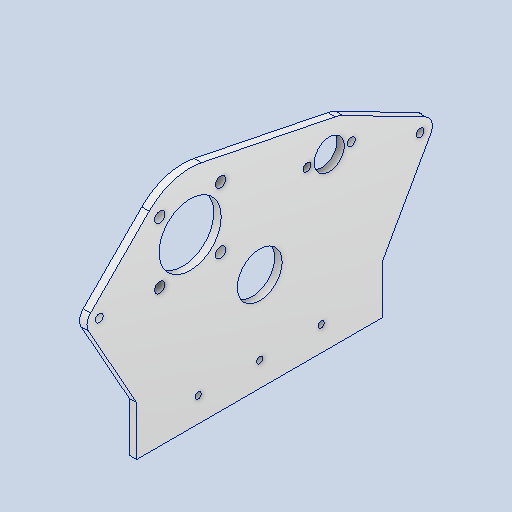
# Autodesk Inventor part: base_weel-v3-Plate-2
Saved by Autodesk Inventor 2025.2 (Build 292293000, 293)
## iProperties
Created: 2025-04-01
Part Number: base_weel-v3-Plate-2
Material: アルミニウム 6061
Document SubType Name: Modeling
Designer: haruy
Density: 2.7 g/cm^3
Appearance: アルミニウム - フラット
Author: haruy
Autodesk Inventor part; units mm, degrees
ref_plane "YZ Plane" through (0, 0, 0) normal (1, 0, 0) x (0, 1, 0)
ref_plane "XZ Plane" through (0, 0, 0) normal (0, 1, 0) x (-1, 0, 0)
ref_plane "XY Plane" through (0, 0, 0) normal (0, 0, 1) x (1, 0, 0)
derived "base_weel-v3-Plate-1.ipt"
sketch "スケッチ1" plane through (0, 0, 0) normal (1, 0, 0) x (0, 1, 0)
  line L0 (0, 0) -> (20, 0)
  line L1 (20, 0) -> (20, -110)
  line L2 (20, -110) -> (0, -110)
  line L3 (0, -110) -> (0, 0)
  circle A0 centre (40, -55) radius 52.5
  line L4 (-12.5, 72.5213) -> (-12.5, -343.3137)
  circle A1 centre (40, -55) radius 9.5 construction
  circle A2 centre (40, -55) radius 20
  circle A3 centre (68.2843, -26.7157) radius 20
  circle A4 centre (68.2843, -83.2843) radius 20
  line L5 (68.2843, -26.7157) -> (40, -55)
  line L6 (40, -55) -> (68.2843, -83.2843)
  line L7 (40, -55) -> (40, -2.5)
  line L8 (0, 15) -> (20, 15)
  line L9 (20, 15) -> (20, -125)
  line L10 (20, -125) -> (0, -125)
  line L11 (0, -125) -> (0, 15)
  circle A5 centre (68.2843, -26.7157) radius 23.5
  circle A6 centre (57.4091, 10.2164) radius 5
  circle A7 centre (57.4091, -120.2164) radius 5
  line L12 (20, -20) -> (0, -20)
  line L13 (0, -55) -> (20, -55)
  circle A8 centre (40, -55) radius 9.1
  circle A9 centre (57.4091, 10.2164) radius 1.6
  circle A10 centre (57.4091, -120.2164) radius 1.6
  line L14 (20, -20) -> (53.8799, 13.7583)
  line L15 (62.4057, 10.0326) -> (59.9865, -55.7352)
  circle A11 centre (10, -55) radius 1.25
  circle A12 centre (10, -35) radius 1.25 construction
  line L16 (62.4057, -120.0326) -> (59.9865, -54.2648)
  line L17 (20, -90) -> (53.8799, -123.7583)
  circle A13 centre (10, -75) radius 1.25 construction
  line L18 (20, -90) -> (0, -90)
  line L19 (20, -5) -> (0, -5)
  circle A14 centre (10, -30) radius 1.25
  circle A15 centre (68.2843, -26.7157) radius 12.6
  circle A16 centre (68.2843, -26.7157) radius 17.5
  circle A17 centre (80.6586, -14.3414) radius 2.1
  line L20 (68.2843, -26.7157) -> (68.2843, -9.2157)
  line L21 (68.2843, -26.7157) -> (80.6586, -14.3414)
  circle A18 centre (55.9099, -14.3414) radius 2.1
  circle A19 centre (55.9099, -39.0901) radius 2.1
  circle A20 centre (80.6586, -39.0901) radius 2.1
  circle A21 centre (68.2843, -83.2843) radius 6.1
  circle A22 centre (68.2843, -83.2843) radius 9
  circle A23 centre (68.2843, -74.2843) radius 1.6
  line L22 (68.2843, -83.2843) -> (68.2843, -74.2843)
  line L23 (20, -5) -> (54.9662, 14.579)
  line L24 (60.9367, 13.7597) -> (84.8644, -10.0619)
  circle A24 centre (68.2843, -83.2843) radius 12.25
  circle A25 centre (68.2843, -92.2843) radius 1.6
  line L25 (91.3149, -31.3893) -> (80.2896, -85.7205)
  line L26 (61.8537, -122.5067) -> (79.1735, -88.8955)
  line L27 (20, -105) -> (0, -105)
  circle A26 centre (10, -80) radius 1.25
  line L28 (20, -105) -> (54.9662, -124.579)
  point P0 (58.8173, -48.2245)
  point P1 (60.2417, -48.7967)
  point P2 (60.6843, -36.7656)
  point P3 (60.4778, -42.3781)
  point P4 (57.4812, -40.4833)
  point P5 (57.3948, -37.6052)
  point P6 (59.3747, -35.6253)
  point P7 (0.8688, -20)
  point P8 (0, -20.9963)
  point P9 (0, -89.0037)
  point P10 (0.8688, -90)
  point P11 (0, -90)
  point P12 (0, -105)
  point P13 (89.8597, -38.5603)
  point P14 (89.359, -37.1131)
  point P15 (0, -5)
  point P16 (0, -20)
  point P17 (60.0135, -55)
  dimension "d14" = 18
  dimension "d1" = 20
  dimension "d2" = 2.5
  dimension "d3" = 25
  dimension "d4" = 10
  dimension "d5" = 25.2
  dimension "d6" = 35
  dimension "d7" = 4.2
  dimension "d8" = 45
  dimension "d11" = 360
  dimension "d13" = 12.2
  dimension "d15" = 3.2
  dimension "d16" = 24.5
  dimension "d19" = 360
  measures "d1" distance between parallel lines of L8 L19
  measures "d2" diameter of A14
  measures "d3" distance from line of A14.centre L13
  measures "d4" distance from line of A14.centre L3
  measures "d5" diameter of A15
  measures "d6" diameter of A16
  measures "d7" diameter of A17
  measures "d13" diameter of A21
  measures "d15" diameter of A23
  measures "d16" diameter of A24
extrude "押し出し1" add sketch "スケッチ1" against normal blind 3 contours L19 L1 A0 L12 L3 | L23 A6 L14 A0 L1 | L12 A0 L3 | A0 L14 L1 | L1 L12 A0 | A6 | A0 L12 L1 L13 A11 L3 | L14 A0 L7 A2 L1 | L14 A6 L15 A5 A0 | L24 A5 L15 A6 | L13 A11 L1 L18 A0 L3 | A2 A4 L16 A0 L17 L1 | A2 L7 A8 L6 | A0 A5 A2 L7 | A5 A0 A3 L15 | A0 L18 L3 | L17 A0 L1 | L1 A0 L18 | A2 A5 L5 A8 L7 | L6 A8 L5 A5 A2 | A2 L15 L16 A4 | L6 A24 L16 A4 | A4 L16 A24 L6 | A5 L15 A0 | A0 L15 A3 A2 A5 | L18 A0 L1 L27 L3 | A0 L17 A7 L28 L1 | A0 L16 A7 L17 | A2 L5 A5 | A2 L16 L15 | L16 L15 A5 A0 L25 A4 | A4 L25 A24 L16 | L16 A24 L26 A0 A4 | A4 A0 L16 | A24 L16 L6 | L6 L16 A22 A24 | A0 A3 L15 | L25 A0 A5 | A0 A4 L26 A7 L16 | A7 | A3 L15 A5 A2 | L5 A19 A16 L15 A3 | A3 L15 A16 A18 A19 L5 | A2 A5 L5 | L16 A2 A5 L15 | A24 L16 A22 A25 A23 L6 | A0 L26 A4 | L6 A22 L16 | A3 A0 A16 A17 | A0 A16 L15 A3 | A5 L15 A3 A0 | L15 A16 A20 A0 A3 | A22 L16 | L16 A22 L6 A21 L22 A23 A25 | A22 A23 L22 A21 L6 | A16 L20 A0 | A0 L20 A15 L15 A16 | L15 A15 L5 A19 A16 A18 | A16 A19 L5 A15 L15 | L15 A15 A0 A16 A20 | L20 A16 A17 L21 A15 A0 | A0 A15 L20 | A0 A15 L21 A17 A16 picked at (71.0949, -99.3068)
